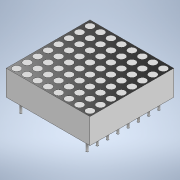
# Autodesk Inventor part: Part6
Saved by Autodesk Inventor 2021 (Build 250183000, 183)
## iProperties
Created: 2023-04-01
Part Number: Part6
Material: Generic
Document SubType Name: Modeling
Designer: stepa
Density: 1 g/cm^3
Appearance: Default
Author: stepa
Autodesk Inventor part; units mm, degrees
ref_plane "YZ Plane" through (0, 0, 0) normal (1, 0, 0) x (0, 1, 0)
ref_plane "XZ Plane" through (0, 0, 0) normal (0, 1, 0) x (-1, 0, 0)
ref_plane "XY Plane" through (0, 0, 0) normal (0, 0, 1) x (1, 0, 0)
sketch "Sketch1" plane through (0, 0, 0) normal (0, 1, 0) x (-1, 0, 0)
  line L0 (10, 10) -> (-10, 10)
  line L1 (-10, 10) -> (-10, -10)
  line L2 (-10, -10) -> (10, -10)
  line L3 (10, -10) -> (10, 10)
  line L4 (10, 10) -> (-10, -10) construction
  line L5 (-10, 10) -> (10, -10) construction
  point P0 (0, 0)
  dimension "d0" = 20
  dimension "d1" = 20
  constraints: 12 end point, 2 midpoint, 2 parallel, 1 horizontal, 1 perpendicular
  measures "d0" distance of L2.end L0.start
  measures "d1" distance of L1.end L2.end
extrude "Extrusion1" add sketch "Sketch1" along normal blind 6
sketch "Sketch2" plane through (0, 6, 0) normal (0, 1, 0) x (1, 0, 0)
  circle A0 centre (8.8, -8.8) radius 0.9
  line L0 (10, -10) -> (10, 10) projected
  line L1 (-10, -10) -> (10, -10) projected
  circle A1 centre (8.8, -6.3) radius 0.9
  circle A2 centre (8.8, -3.8) radius 0.9
  circle A3 centre (8.8, -1.3) radius 0.9
  circle A4 centre (8.8, 1.2) radius 0.9
  circle A5 centre (8.8, 3.7) radius 0.9
  circle A6 centre (8.8, 6.2) radius 0.9
  circle A7 centre (8.8, 8.7) radius 0.9
  circle A8 centre (6.3, -8.8) radius 0.9
  circle A9 centre (6.3, -6.3) radius 0.9
  circle A10 centre (6.3, -3.8) radius 0.9
  circle A11 centre (6.3, -1.3) radius 0.9
  circle A12 centre (6.3, 1.2) radius 0.9
  circle A13 centre (6.3, 3.7) radius 0.9
  circle A14 centre (6.3, 6.2) radius 0.9
  circle A15 centre (6.3, 8.7) radius 0.9
  circle A16 centre (3.8, -8.8) radius 0.9
  circle A17 centre (3.8, -6.3) radius 0.9
  circle A18 centre (3.8, -3.8) radius 0.9
  circle A19 centre (3.8, -1.3) radius 0.9
  circle A20 centre (3.8, 1.2) radius 0.9
  circle A21 centre (3.8, 3.7) radius 0.9
  circle A22 centre (3.8, 6.2) radius 0.9
  circle A23 centre (3.8, 8.7) radius 0.9
  circle A24 centre (1.3, -8.8) radius 0.9
  circle A25 centre (1.3, -6.3) radius 0.9
  circle A26 centre (1.3, -3.8) radius 0.9
  circle A27 centre (1.3, -1.3) radius 0.9
  circle A28 centre (1.3, 1.2) radius 0.9
  circle A29 centre (1.3, 3.7) radius 0.9
  circle A30 centre (1.3, 6.2) radius 0.9
  circle A31 centre (1.3, 8.7) radius 0.9
  circle A32 centre (-1.2, -8.8) radius 0.9
  circle A33 centre (-1.2, -6.3) radius 0.9
  circle A34 centre (-1.2, -3.8) radius 0.9
  circle A35 centre (-1.2, -1.3) radius 0.9
  circle A36 centre (-1.2, 1.2) radius 0.9
  circle A37 centre (-1.2, 3.7) radius 0.9
  circle A38 centre (-1.2, 6.2) radius 0.9
  circle A39 centre (-1.2, 8.7) radius 0.9
  circle A40 centre (-3.7, -8.8) radius 0.9
  circle A41 centre (-3.7, -6.3) radius 0.9
  circle A42 centre (-3.7, -3.8) radius 0.9
  circle A43 centre (-3.7, -1.3) radius 0.9
  circle A44 centre (-3.7, 1.2) radius 0.9
  circle A45 centre (-3.7, 3.7) radius 0.9
  circle A46 centre (-3.7, 6.2) radius 0.9
  circle A47 centre (-3.7, 8.7) radius 0.9
  circle A48 centre (-6.2, -8.8) radius 0.9
  circle A49 centre (-6.2, -6.3) radius 0.9
  circle A50 centre (-6.2, -3.8) radius 0.9
  circle A51 centre (-6.2, -1.3) radius 0.9
  circle A52 centre (-6.2, 1.2) radius 0.9
  circle A53 centre (-6.2, 3.7) radius 0.9
  circle A54 centre (-6.2, 6.2) radius 0.9
  circle A55 centre (-6.2, 8.7) radius 0.9
  circle A56 centre (-8.7, -8.8) radius 0.9
  circle A57 centre (-8.7, -6.3) radius 0.9
  circle A58 centre (-8.7, -3.8) radius 0.9
  circle A59 centre (-8.7, -1.3) radius 0.9
  circle A60 centre (-8.7, 1.2) radius 0.9
  circle A61 centre (-8.7, 3.7) radius 0.9
  circle A62 centre (-8.7, 6.2) radius 0.9
  circle A63 centre (-8.7, 8.7) radius 0.9
  point P0 (0, 0)
  dimension "d4" = 1.8
  dimension "d5" = 1.2
  dimension "d6" = 1.2
  dimension "d9" = 2.5
  dimension "d12" = 2.5
  constraints: 64 centre point, 1 horizontal, 1 vertical, 126 other
  measures "d4" diameter of A0
  measures "d5" distance from line of L0 A0.centre
  measures "d6" distance from line of L1 A0.centre
  measures "d9" distance of A0.centre A1.centre
  measures "d12" distance of A0.centre A8.centre
extrude "Extrusion2" cut sketch "Sketch2" against normal blind 0.005 contours A0
pattern_linear "Rectangular Pattern1" count 8 spacing 2.5 along (-1, 0, 0) count 8 spacing 2.5 along (0, 0, -1) of "Extrusion2"
sketch "Sketch3" plane through (0, 0, 0) normal (0, -1, 0) x (1, 0, 0)
  circle A0 centre (-8, 8.5) radius 0.25
  line L0 (-10, 10) -> (10, 10) projected
  line L1 (10, 10) -> (10, -10) projected
  line L2 (10, -10) -> (-10, -10) projected
  line L3 (-10, -10) -> (-10, 10) projected
  point P0 (0, 0)
  dimension "d23" = 0.5
  dimension "d24" = 1.5
  dimension "d25" = 2
  constraints: 1 centre point
  measures "d23" diameter of A0
  measures "d24" distance from line of L0 A0.centre
  measures "d25" distance from line of L3 A0.centre
extrude "Extrusion3" add sketch "Sketch3" along normal blind 3 contours A0
pattern_linear "Rectangular Pattern2" count 8 spacing 2.45 along (0, 0, -1) count 2 spacing 15.8 along (1, 0, 0) of "Extrusion3"
body "Solid1"
